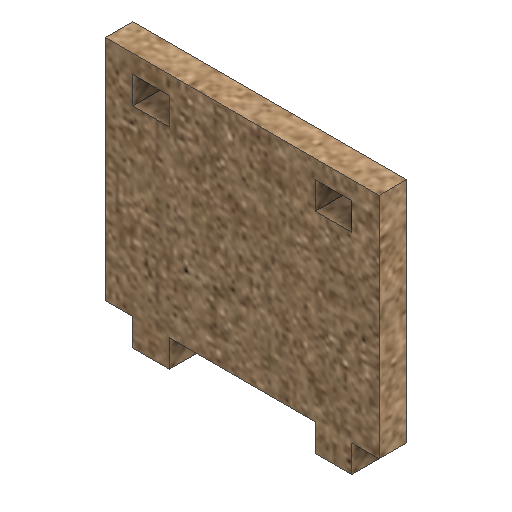
# Autodesk Inventor part: test_side_hold_2
Saved by Autodesk Inventor 2024 (Build 280153000, 153)
## iProperties
Created: 2024-05-27
Part Number: test_side_hold_2
Material: MDF Medium Density Fiberboard
Document SubType Name: Modeling
Designer: op04o
Density: 0.8 g/cm^3
Appearance: Cardboard - Corrugated
Mass: 1.8 g
Surface Area: 19.5 cm^2
Volume: 2.25 cm^3
Author: op04o
Autodesk Inventor part; units mm, degrees
ref_plane "YZ Plane" through (0, 0, 0) normal (1, 0, 0) x (0, 1, 0)
ref_plane "XZ Plane" through (0, 0, 0) normal (0, 1, 0) x (-1, 0, 0)
ref_plane "XY Plane" through (0, 0, 0) normal (0, 0, 1) x (1, 0, 0)
sketch "Sketch1" plane through (0, 0, 0) normal (0, 0, 1) x (1, 0, 0)
  line L0 (-15, 12.5) -> (15, 12.5)
  line L1 (15, 12.5) -> (15, -12.5)
  line L2 (15, -12.5) -> (-15, -12.5)
  line L3 (-15, -12.5) -> (-15, 12.5)
  line L4 (-12, 10.5) -> (-8, 10.5)
  line L5 (-8, 10.5) -> (-8, 7.5)
  line L6 (-8, 7.5) -> (-12, 7.5)
  line L7 (-12, 7.5) -> (-12, 10.5)
  line L8 (8, 10.5) -> (12, 10.5)
  line L9 (12, 10.5) -> (12, 7.5)
  line L10 (12, 7.5) -> (8, 7.5)
  line L11 (8, 7.5) -> (8, 10.5)
  line L12 (-12, -12.5) -> (-8, -12.5)
  line L13 (-8, -12.5) -> (-8, -15.5)
  line L14 (-8, -15.5) -> (-12, -15.5)
  line L15 (-12, -15.5) -> (-12, -12.5)
  line L16 (8, -12.5) -> (12, -12.5)
  line L17 (12, -12.5) -> (12, -15.5)
  line L18 (12, -15.5) -> (8, -15.5)
  line L19 (8, -15.5) -> (8, -12.5)
  point P0 (0, 0)
  point P1 (0, 12.5)
  point P2 (15, 0)
  point P3 (-10, -12.5)
  point P4 (0, -12.5)
  point P5 (10, -12.5)
  point P6 (-10, 10.5)
  point P7 (10, 10.5)
  dimension "d0" = 25
  dimension "d1" = 30
  dimension "d2" = 4
  dimension "d3" = 3
  dimension "d4" = 3
  dimension "d5" = 4
  dimension "d6" = 10
  dimension "d7" = 10
  dimension "d8" = 10
  dimension "d9" = 10
  dimension "d10" = 20
  constraints: 40 end point, 10 parallel, 7 midpoint, 5 horizontal, 5 perpendicular, 5 point on line, 2 collinear, 1 horizontal alignment, 1 vertical alignment
  measures "d0" distance of L0.end L1.end
  measures "d1" distance of L1.end L2.end
  measures "d2" distance of L4.start L4.end
  measures "d3" distance of L6.end L4.start
  measures "d4" distance of L14.end L12.start
  measures "d5" distance of L13.end L14.end
  measures "d6" distance of point (-10, -12.5) point (0, -12.5)
  measures "d7" distance of point (0, -12.5) point (10, -12.5)
  measures "d8" horizontal distance of point (0, 12.5) point (-10, 10.5)
  measures "d9" horizontal distance of point (0, 12.5) point (10, 10.5)
  measures "d10" distance between parallel lines of L2 L10
extrude "Extrusion1" add sketch "Sketch1" along normal blind 3
body "Solid1"
